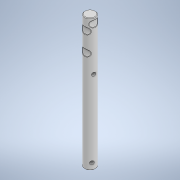
# Autodesk Inventor part: 80. Шток заднего хода
Saved by Autodesk Inventor 2021 (Build 250183000, 183)
## iProperties
Created: 2021-03-18
Part Number: 80. Шток заднего хода
Material: Типовые
Document SubType Name: Modeling
Designer: Данил
Density: 1 g/cm^3
Appearance: По умолчанию
Author: Данил
Autodesk Inventor part; units mm, degrees
ref_plane "YZ Plane" through (0, 0, 0) normal (1, 0, 0) x (0, 1, 0)
sketch "Эскиз1" plane through (0, 0, 0) normal (0, 0, 1) x (1, 0, 0)
  line L0 (0, 91.5) -> (0, -91.5)
  line L1 (0, -91.5) -> (6.75, -91.5)
  line L2 (7.5, -90.75) -> (7.5, 90.75)
  line L3 (7.5, -90.75) -> (6.75, -91.5)
  line L4 (6.75, 91.5) -> (0, 91.5)
  line L5 (7.5, 90.75) -> (6.75, 91.5)
  point P0 (0, 0)
  point P1 (0, 0)
  point P2 (7.5, -91.5)
  point P3 (7.5, 91.5)
  dimension "d0" = 183
  dimension "d1" = 0.75
  dimension "d2" = 45
  dimension "d3" = 15
  dimension "d10" = 0.75
  dimension "d11" = 45
  constraints: 12 end point, 4 point on line, 2 horizontal, 1 coincident, 1 midpoint, 1 perpendicular, 1 vertical
  measures "d0" distance of L0.start L0.end
  measures "d1" distance of L2.start point (7.5, -91.5)
  measures "d2" angle of L2 L3
  measures "d3" diameter of L2 L0
  measures "d10" distance of L2.end point (7.5, 91.5)
  measures "d11" angle of L2 L5
revolve "Вращение1" add sketch "Эскиз1" angle 360 about axis through (0, 91.5, 0) along (0, -1, 0)
sketch "Эскиз2" plane through (0, 0, 0) normal (0, 0, 1) x (1, 0, 0)
  line L0 (7.5, 90.75) -> (7.5, -90.75) projected
  line L1 (-7.5, 90.75) -> (-7.5, -90.75) projected
  arc A0 (7.5, 88.5) -> (7.5, 79.6006) centre (9.3, 84.0503) ccw
  line L2 (-6.75, 91.5) -> (6.75, 91.5) projected
  point P0 (0, 0)
  point P1 (4.5, 84.0503)
  dimension "d13" = 4.8
  dimension "d14" = 3
  dimension "d15" = 12
  constraints: 3 point on circle, 2 point on line, 1 centre point, 1 horizontal alignment
  measures "d13" radius of A0
  measures "d14" distance from line of L2 A0.start
  measures "d15" distance from line of L1 point (4.5, 84.05)
extrude "Выдавливание1" cut sketch "Эскиз2" against normal through all both and the other way through all
fillet "Сопряжение1" radius 0.8 2 edges at (4.5, 84.0509, 6) (4.5, 84.0509, -6)
sketch "Эскиз3" plane through (0, 0, 0) normal (1, 0, 0) x (0, 1, 0)
  arc A0 (71.1872, 7.5) -> (79.8128, 7.5) centre (75.5, 9.1) ccw
  line L0 (90.75, 7.5) -> (-90.75, 7.5) projected
  line L1 (91.5, 6.75) -> (91.5, -6.75) projected
  line L2 (90.75, -7.5) -> (-90.75, -7.5) projected
  point P0 (0, 0)
  point P1 (75.5, 4.5)
  dimension "d19" = 4.6
  dimension "d21" = 16
  dimension "d22" = 12
  constraints: 3 point on circle, 2 point on line, 1 centre point, 1 vertical alignment
  measures "d19" radius of A0
  measures "d21" distance from line of L1 A0.centre
  measures "d22" distance from line of L2 point (75.5, 4.5)
extrude "Выдавливание2" cut sketch "Эскиз3" against normal through all both and the other way through all
fillet "Сопряжение2" radius 0.8 2 edges at (-6, 75.5052, 4.5) (6, 75.5043, 4.5)
pattern_linear "Прямоуг.массив1" count 2 spacing 26.5 along (0, -1, 0) of "Выдавливание2", "Сопряжение2"
ref_plane "РабПлоскость1" through (0, 23.5, 0) normal (0, 1, 0) x (1, 0, 0)
sketch "Эскиз4" plane through (0, 23.5, 0) normal (0, 1, 0) x (1, 0, 0)
  line L0 (9.6593, -2.5882) -> (-9.6593, 2.5882)
  circle A0 centre (0, 0) radius 7.5 projected
  line L1 (7.5, 0) -> (-7.5, 0) construction
  line L2 (-9.6593, 2.5882) -> (-9.0122, 5.003)
  line L3 (-9.0122, 5.003) -> (10.3063, -0.1734)
  line L4 (10.3063, -0.1734) -> (9.6593, -2.5882)
  point P0 (0, 0)
  point P1 (0, 0)
  dimension "d30" = 15
  dimension "d31" = 20
  dimension "d32" = 5
  constraints: 10 end point, 2 midpoint, 2 perpendicular, 2 point on circle, 1 coincident, 1 horizontal, 1 parallel
  measures "d30" angle of L1 L0
  measures "d31" distance of L0.start L0.end
  measures "d32" diameter of L3 L0
revolve "Вращение2" cut sketch "Эскиз4" angle 360 about axis through (9.6593, 23.5, 2.5882) along (-0.9659258, 0, -0.258819) contours L0 A0 L3 L4 | L0 A0 L3 | L0 L2 L3 A0
ref_plane "РабПлоскость2" through (0, -82.5, 0) normal (0, 1, 0) x (1, 0, 0)
sketch "Эскиз5" plane through (0, -82.5, 0) normal (0, 1, 0) x (1, 0, 0)
  circle A0 centre (0, 0) radius 7.5 projected
  line L0 (7.5, 0) -> (-7.5, 0) construction
  line L1 (-8.6603, 5) -> (8.6603, -5)
  line L2 (-8.6603, 5) -> (-7.4103, 7.1651)
  line L3 (-7.4103, 7.1651) -> (9.9103, -2.8349)
  line L4 (9.9103, -2.8349) -> (8.6603, -5)
  point P0 (0, 0)
  point P1 (0, 0)
  dimension "d35" = 30
  dimension "d36" = 20
  dimension "d37" = 5
  constraints: 10 end point, 2 midpoint, 2 perpendicular, 2 point on circle, 1 coincident, 1 horizontal
  measures "d35" angle of L0 L1
  measures "d36" distance of L1.start L1.end
  measures "d37" diameter of L3 L1
revolve "Вращение3" cut sketch "Эскиз5" angle 360 about axis through (-8.6603, -82.5, -5) along (0.8660254, 0, 0.5) contours L3 A0 L1 | A0 L1 L2 L3 | L3 L4 L1 A0
